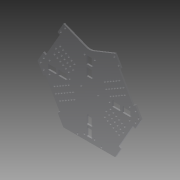
# Autodesk Inventor part: Bottom Plate
Saved by Autodesk Inventor 2015 (Build 190159000, 159)
## iProperties
Created: 2015-11-27
Part Number: Bottom Plate
Material: Polycarbonate, Clear
Document SubType Name: Modeling
Designer: James
Density: 1.2 g/cm^3
Appearance: Polycarbonate - Clear
Author: James
Autodesk Inventor part; units mm, degrees
ref_plane "YZ Plane" through (0, 0, 0) normal (1, 0, 0) x (0, 1, 0)
ref_plane "XZ Plane" through (0, 0, 0) normal (0, 1, 0) x (-1, 0, 0)
ref_plane "XY Plane" through (0, 0, 0) normal (0, 0, 1) x (1, 0, 0)
sketch "Sketch1" plane through (0, 0, 0) normal (0, 1, 0) x (-1, 0, 0)
  circle A0 centre (65.1273, -37.6013) radius 1.65
  circle A1 centre (59.628, -34.4263) radius 1.65
  circle A2 centre (54.1288, -31.2513) radius 1.65
  circle A3 centre (48.6295, -28.0763) radius 1.65
  circle A4 centre (43.1303, -24.9013) radius 1.65
  circle A5 centre (37.631, -21.7263) radius 1.65
  circle A6 centre (32.1317, -18.5513) radius 1.65
  circle A7 centre (29.5213, -29.5726) radius 1.7
  circle A8 centre (35.0206, -32.7476) radius 1.7
  circle A9 centre (40.5198, -35.9226) radius 1.7
  circle A10 centre (46.0191, -39.0976) radius 1.7
  circle A11 centre (51.5184, -42.2726) radius 1.7
  circle A12 centre (57.0176, -45.4476) radius 1.7
  circle A13 centre (67.8676, -26.6549) radius 1.7
  circle A14 centre (62.3684, -23.4799) radius 1.7
  circle A15 centre (56.8691, -20.3049) radius 1.7
  circle A16 centre (51.3698, -17.1299) radius 1.7
  circle A17 centre (45.8706, -13.9549) radius 1.7
  circle A18 centre (40.3713, -10.7799) radius 1.7
  line L0 (-70.6699, 40.8013) -> (-56.9199, 64.617)
  line L1 (-70.6699, 40.8013) -> (-84.4199, 16.9856)
  line L2 (-84.4199, 16.9856) -> (-88.75, 19.4856)
  line L3 (-56.9199, 64.617) -> (-61.25, 67.117)
  circle A19 centre (-65.1273, 37.6013) radius 1.65
  circle A20 centre (-59.628, 34.4263) radius 1.65
  circle A21 centre (-54.1288, 31.2513) radius 1.65
  circle A22 centre (-48.6295, 28.0763) radius 1.65
  circle A23 centre (-43.1303, 24.9013) radius 1.65
  circle A24 centre (-37.631, 21.7263) radius 1.65
  circle A25 centre (-32.1317, 18.5513) radius 1.65
  circle A26 centre (-29.5213, 29.5726) radius 1.7
  circle A27 centre (-35.0206, 32.7476) radius 1.7
  circle A28 centre (-40.5198, 35.9226) radius 1.7
  circle A29 centre (-46.0191, 39.0976) radius 1.7
  circle A30 centre (-51.5184, 42.2726) radius 1.7
  circle A31 centre (-57.0176, 45.4476) radius 1.7
  circle A32 centre (-67.8676, 26.6549) radius 1.7
  circle A33 centre (-62.3684, 23.4799) radius 1.7
  circle A34 centre (-56.8691, 20.3049) radius 1.7
  circle A35 centre (-51.3698, 17.1299) radius 1.7
  circle A36 centre (-45.8706, 13.9549) radius 1.7
  circle A37 centre (-40.3713, 10.7799) radius 1.7
  line L4 (70.6699, 40.8013) -> (84.4199, 16.9856)
  line L5 (70.6699, 40.8013) -> (56.9199, 64.617)
  line L6 (56.9199, 64.617) -> (61.25, 67.117)
  line L7 (84.4199, 16.9856) -> (88.75, 19.4856)
  circle A38 centre (65.1273, 37.6013) radius 1.65
  circle A39 centre (59.628, 34.4263) radius 1.65
  circle A40 centre (54.1288, 31.2513) radius 1.65
  circle A41 centre (48.6295, 28.0763) radius 1.65
  circle A42 centre (43.1303, 24.9013) radius 1.65
  circle A43 centre (37.631, 21.7263) radius 1.65
  circle A44 centre (32.1317, 18.5513) radius 1.65
  circle A45 centre (40.3713, 10.7799) radius 1.7
  circle A46 centre (45.8706, 13.9549) radius 1.7
  circle A47 centre (51.3698, 17.1299) radius 1.7
  circle A48 centre (56.8691, 20.3049) radius 1.7
  circle A49 centre (62.3684, 23.4799) radius 1.7
  circle A50 centre (67.8676, 26.6549) radius 1.7
  circle A51 centre (57.0176, 45.4476) radius 1.7
  circle A52 centre (51.5184, 42.2726) radius 1.7
  circle A53 centre (46.0191, 39.0976) radius 1.7
  circle A54 centre (40.5198, 35.9226) radius 1.7
  circle A55 centre (35.0206, 32.7476) radius 1.7
  circle A56 centre (29.5213, 29.5726) radius 1.7
  line L8 (-88.75, -19.4856) -> (-84.4199, -16.9856)
  line L9 (-84.4199, -16.9856) -> (-56.9199, -64.617)
  line L10 (-56.9199, -64.617) -> (-61.25, -67.117)
  line L11 (61.25, -67.117) -> (56.9199, -64.617)
  line L12 (56.9199, -64.617) -> (84.4199, -16.9856)
  line L13 (84.4199, -16.9856) -> (88.75, -19.4856)
  circle A57 centre (-65.1273, -37.6013) radius 1.65
  circle A58 centre (-59.628, -34.4263) radius 1.65
  circle A59 centre (-54.1288, -31.2513) radius 1.65
  circle A60 centre (-48.6295, -28.0763) radius 1.65
  circle A61 centre (-43.1303, -24.9013) radius 1.65
  circle A62 centre (-37.631, -21.7263) radius 1.65
  circle A63 centre (-32.1317, -18.5513) radius 1.65
  circle A64 centre (-40.3713, -10.7799) radius 1.7
  circle A65 centre (-45.8706, -13.9549) radius 1.7
  circle A66 centre (-51.3698, -17.1299) radius 1.7
  circle A67 centre (-56.8691, -20.3049) radius 1.7
  circle A68 centre (-62.3684, -23.4799) radius 1.7
  circle A69 centre (-67.8676, -26.6549) radius 1.7
  circle A70 centre (-57.0176, -45.4476) radius 1.7
  circle A71 centre (-51.5184, -42.2726) radius 1.7
  circle A72 centre (-46.0191, -39.0976) radius 1.7
  circle A73 centre (-40.5198, -35.9226) radius 1.7
  circle A74 centre (-35.0206, -32.7476) radius 1.7
  circle A75 centre (-29.5213, -29.5726) radius 1.7
  line L14 (-88.75, 19.4856) -> (-100, 0)
  line L15 (-100, 0) -> (-88.75, -19.4856)
  line L16 (-61.25, -67.117) -> (-50, -86.6025)
  line L17 (-50, -86.6025) -> (50, -86.6025)
  line L18 (50, -86.6025) -> (61.25, -67.117)
  line L19 (88.75, -19.4856) -> (100, 0)
  line L20 (100, 0) -> (88.75, 19.4856)
  line L21 (61.25, 67.117) -> (50, 86.6025)
  line L22 (-50, 86.6025) -> (-61.25, 67.117)
  circle A76 centre (88.75, -9.7428) radius 1.6
  circle A77 centre (88.75, 9.7428) radius 1.6
  circle A78 centre (94.375, 0) radius 1.6
  circle A79 centre (-88.75, -9.7428) radius 1.6
  circle A80 centre (-88.75, 9.7428) radius 1.6
  circle A81 centre (-94.375, 0) radius 1.6
  line L23 (-56.9199, 64.617) -> (-61.25, 67.117)
  line L24 (56.9199, 64.617) -> (61.25, 67.117)
  line L25 (61.25, 67.117) -> (50, 86.6025)
  line L26 (-50, 86.6025) -> (-61.25, 67.117)
  circle A82 centre (-47.5441, 80.2626) radius 1.6
  circle A83 centre (-55.9574, 69.7681) radius 1.6
  circle A84 centre (47.5441, 80.2626) radius 1.6
  circle A85 centre (55.9574, 69.7681) radius 1.6
  line L27 (0, 56.6025) -> (-5, 56.6025)
  line L28 (-5, 56.6025) -> (-5, 46.6025)
  line L29 (-5, 46.6025) -> (-5, 41.6025)
  line L30 (-5, 41.6025) -> (5, 41.6025)
  line L31 (5, 41.6025) -> (5, 56.6025)
  line L32 (5, 56.6025) -> (0, 56.6025)
  line L33 (0, 36.6025) -> (-5, 36.6025)
  line L34 (-5, 36.6025) -> (-5, 26.6025)
  line L35 (-5, 26.6025) -> (-5, 21.6025)
  line L36 (-5, 21.6025) -> (5, 21.6025)
  line L37 (5, 21.6025) -> (5, 36.6025)
  line L38 (5, 36.6025) -> (0, 36.6025)
  line L39 (0, -43.6025) -> (-5, -43.6025)
  line L40 (-5, -43.6025) -> (-5, -53.6025)
  line L41 (-5, -53.6025) -> (-5, -58.6025)
  line L42 (-5, -58.6025) -> (5, -58.6025)
  line L43 (5, -58.6025) -> (5, -43.6025)
  line L44 (5, -43.6025) -> (0, -43.6025)
  line L45 (0, -63.6025) -> (-5, -63.6025)
  line L46 (-5, -63.6025) -> (-5, -73.6025)
  line L47 (-5, -73.6025) -> (-5, -78.6025)
  line L48 (-5, -78.6025) -> (5, -78.6025)
  line L49 (5, -78.6025) -> (5, -63.6025)
  line L50 (5, -63.6025) -> (0, -63.6025)
  line L51 (-44.4199, 0) -> (-44.4199, 5)
  line L52 (-44.4199, 5) -> (-54.4199, 5)
  line L53 (-54.4199, 5) -> (-59.4199, 5)
  line L54 (-59.4199, 5) -> (-59.4199, -5)
  line L55 (-59.4199, -5) -> (-44.4199, -5)
  line L56 (-44.4199, -5) -> (-44.4199, 0)
  line L57 (-64.4199, 0) -> (-64.4199, 5)
  line L58 (-64.4199, 5) -> (-74.4199, 5)
  line L59 (-74.4199, 5) -> (-79.4199, 5)
  line L60 (-79.4199, 5) -> (-79.4199, -5)
  line L61 (-79.4199, -5) -> (-64.4199, -5)
  line L62 (-64.4199, -5) -> (-64.4199, 0)
  line L63 (44.4199, 0) -> (44.4199, 5)
  line L64 (44.4199, 5) -> (54.4199, 5)
  line L65 (54.4199, 5) -> (59.4199, 5)
  line L66 (59.4199, 5) -> (59.4199, -5)
  line L67 (59.4199, -5) -> (44.4199, -5)
  line L68 (44.4199, -5) -> (44.4199, 0)
  line L69 (64.4199, 0) -> (64.4199, 5)
  line L70 (64.4199, 5) -> (74.4199, 5)
  line L71 (74.4199, 5) -> (79.4199, 5)
  line L72 (79.4199, 5) -> (79.4199, -5)
  line L73 (79.4199, -5) -> (64.4199, -5)
  line L74 (64.4199, -5) -> (64.4199, 0)
  circle A86 centre (-9.8064, -77.6025) radius 1.6
  circle A87 centre (9.8064, -77.6025) radius 1.6
  circle A88 centre (-16.3064, 0) radius 1.6
  circle A89 centre (16.3064, 0) radius 1.6
  circle A90 centre (-9.8064, 55.6025) radius 1.6
  circle A91 centre (9.8064, 55.6025) radius 1.6
  circle A92 centre (-77.5383, 11.4526) radius 1.6
  circle A93 centre (-77.5383, -11.4526) radius 1.6
  circle A94 centre (-38.7465, 0) radius 1.6
  circle A95 centre (77.5383, 11.4526) radius 1.6
  circle A96 centre (77.5383, -11.4526) radius 1.6
  circle A97 centre (38.7465, 0) radius 1.6
  circle A98 centre (-22.9226, -83.7202) radius 1.6
  circle A99 centre (22.9226, -83.7202) radius 1.6
  line L75 (-7.4278, 69.5737) -> (-50, 86.6025)
  line L76 (7.4278, 69.5737) -> (50, 86.6025)
  arc A100 (-7.4278, 69.5737) -> (7.4278, 69.5737) centre (0, 88.1432) ccw
  constraints: 154 end point, 101 centre point, 8 point on line, 2 point on circle
extrude "Extrusion2" add sketch "Sketch1" along normal blind 3
body "Solid2"
